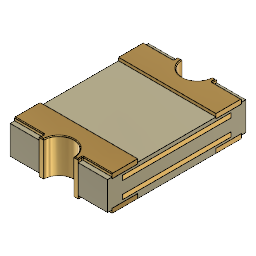
SMD+PTC+Fuse+MF-MSMF250_16X (Autodesk Fusion 360 design; units mm, degrees)
Autodesk Fusion 360 part; units mm, degrees
note: some values were not read from the file. Chosen so that the rebuilt part matches the saved one: which bodies a step acts on; which face or edge a step refers to. Set by a fixed rule: which sketch regions a step uses.
sketch "Sketch1" plane through (0, 0, 0) normal (1, 0, 0) x (0, 1, 0)
  line L0 (-2.3, 1.25) -> (2.3, 1.25)
  line L1 (2.3, 1.25) -> (2.3, 0.1)
  line L2 (2.3, 0.1) -> (-2.3, 0.1)
  line L3 (-2.3, 0.1) -> (-2.3, 1.25)
  line L4 (-1.3, 1.25) -> (-2.15, 1.25)
  line L5 (-2.15, 1.25) -> (-2.15, 1.1)
  line L6 (-2.15, 1.1) -> (-1.3, 1.1)
  line L7 (-1.3, 1.1) -> (-1.3, 1.25)
  line L8 (-2.15, 0.25) -> (-1.3, 0.25)
  line L9 (-1.3, 0.25) -> (-1.3, 0.1)
  line L10 (-1.3, 0.1) -> (-2.15, 0.1)
  line L11 (-2.15, 0.1) -> (-2.15, 0.25)
  line L12 (0, 0) -> (0, 0.1) construction
  line L13 (-2.3, 0.675) -> (-0.9368, 0.675) construction
  line L14 (1.3, 1.25) -> (2.15, 1.25)
  line L15 (2.15, 1.25) -> (2.15, 1.1)
  line L16 (2.15, 1.1) -> (1.3, 1.1)
  line L17 (1.3, 1.1) -> (1.3, 1.25)
  line L18 (1.3, 0.1) -> (2.15, 0.1)
  line L19 (2.15, 0.1) -> (2.15, 0.25)
  line L20 (1.3, 0.25) -> (1.3, 0.1)
  line L21 (2.15, 0.25) -> (1.3, 0.25)
  line L22 (1.8, 0.875) -> (-1.8, 0.875)
  line L23 (-1.8, 0.875) -> (-1.8, 1.025)
  line L24 (-1.8, 1.025) -> (1.8, 1.025)
  line L25 (1.8, 1.025) -> (1.8, 0.875)
  line L26 (1.8, 0.875) -> (-1.8, 1.025) construction
  line L27 (-1.8, 0.875) -> (1.8, 1.025) construction
  line L28 (1.8, 0.475) -> (-1.8, 0.475)
  line L29 (-1.8, 0.475) -> (-1.8, 0.325)
  line L30 (-1.8, 0.325) -> (1.8, 0.325)
  line L31 (1.8, 0.325) -> (1.8, 0.475)
  line L32 (-2.3, 1.15) -> (-2.15, 1.15)
  line L33 (-1.3, 1.15) -> (1.3, 1.15)
  line L34 (2.15, 1.15) -> (2.3, 1.15)
  line L35 (-2.3, 0.2) -> (-2.15, 0.2)
  line L36 (-1.3, 0.2) -> (1.3, 0.2)
  line L37 (2.15, 0.2) -> (2.3, 0.2)
  dimension "d1" = 0.1
  dimension "d2" = 0.15
  dimension "d4" = 0.15
  dimension "d5" = 2.6
  dimension "d6" = 4.6
  dimension "d7" = 1.15
  dimension "d8" = 0.3
  dimension "d9" = 0.5
  dimension "d19" = 0.1
  dimension "d20" = 0.15
  dimension "d21" = 0.15
  measures "d1" distance of L12.start L2
  measures "d2" distance of L8 L10
  measures "d8" distance of L0
  measures "d9" distance of L3
  measures "d19" distance of L0 L32
extrude "Extrude1" add sketch "Sketch1" along normal mid plane 3.24 contours L1 L3 L5 L6 L7 L8 L9 L11 L15 L16 L17 L19 L20 L21 L32 L33 L34 L35 L36 L37 | L2 L9 L20 L36 makes body 1
extrude "Extrude2" add sketch "Sketch1" along normal mid plane 3.24 separate body contours L0 L4 L5 L6 L7 | L0 L14 L15 L16 L17 | L2 L8 L9 L10 L11 | L2 L18 L19 L20 L21 | L22 L23 L24 L25 | L28 L29 L30 L31 makes body 2 at (-0.54, -1.8667, 0.25) makes body 3 at (0.54, -1.5833, 1.25) makes body 4 at (0.54, 1.8667, 1.25) makes body 5 at (0.54, 0.6, 0.325) makes body 6 at (-0.54, -0.6, 1.025) makes body 7 at (0.54, 1.5833, 0.1)
sketch "Sketch2" plane through (0, 0, 1.25) normal (0, 0, 1) x (-1, 0, 0)
  line L0 (-1.62, 2.15) -> (-1.62, 1.3)
  line L1 (-1.62, 1.3) -> (1.62, 1.3)
  line L2 (1.62, 1.3) -> (1.62, 2.15)
  circle A0 centre (0, 2.3) radius 0.5
  circle A1 centre (0, -2.3) radius 0.5
  circle A2 centre (0, 2.3) radius 0.65
  circle A3 centre (0, -2.3) radius 0.65
  line L3 (1.62, -2.3) -> (-1.62, -2.3)
  line L4 (0, 0) -> (-1.3375, 0) construction
  line L5 (1.62, 2.3) -> (-1.62, 2.3)
  dimension "d14" = 1
  dimension "d15" = 0.15
  measures "d14" diameter of A0
  measures "d15" distance of A0 A2
extrude "Extrude3" cut sketch "Sketch2" against normal through all contours A0 A2 L5 | A0 A2 L5 | A0 L5 | A1 L3 | A1 A3 L3 | A1 L3 picked at (-0.1222, 2.1866) picked at (-0.5957, -2.2429) bodies 1 2 4 5 6 3 7
extrude "Extrude4" add sketch "Sketch2" against normal blind 1.15 contours A0 A2 L5 | A1 A3 L3 picked at (-0.5976, 2.2677) picked at (-0.5957, -2.2429) bodies 2 4 3 7
fillet "Fillet1" radius 0.025 18 edges at (-1.1262, -2.15, 1.25) (-0.6456, -2.2245, 1.25) (-0.575, -2.3, 1.25) (0, -1.8, 1.25) (0.575, -2.3, 1.25) (0.6325, -2.15, 1.175) (0.6456, -2.2245, 1.25) (1.1262, -2.15, 1.25) (-0.6325, -2.15, 1.175) (0, 1.8, 1.25) (-0.575, 2.3, 1.25) (-0.6456, 2.2245, 1.25) (-0.6325, 2.15, 1.175) (-1.1262, 2.15, 1.25) (0.575, 2.3, 1.25) (0.6325, 2.15, 1.175) (0.6456, 2.2245, 1.25) (1.1262, 2.15, 1.25) on bodies 2 4
equation "d10 = 3.24 mm"
equation "d12 = d10"
equation "d20 = d2"
